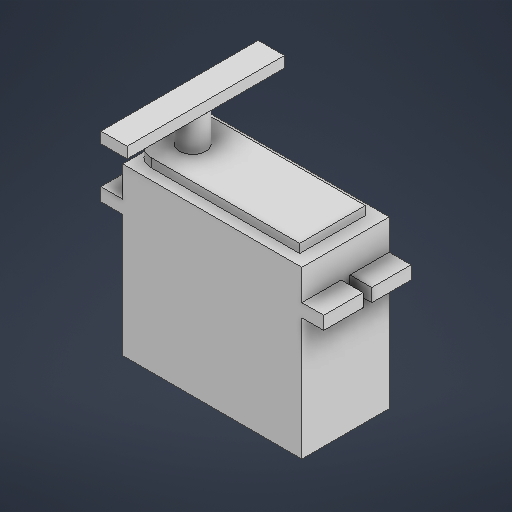
# Autodesk Inventor part: Servomoteur analogique FS5106B
Saved by Autodesk Inventor 2026.2 (Build 302298010, 298A)
## iProperties
Created: 2026-03-17
Part Number: Servomoteur analogique FS5106B
Material: Générique
Document SubType Name: Modeling
Designer: cleml
Density: 1 g/cm^3
Appearance: Par défaut
Author: cleml
Autodesk Inventor part; units mm, degrees
ref_plane "YZ Plane" through (0, 0, 0) normal (1, 0, 0) x (0, 1, 0)
ref_plane "XZ Plane" through (0, 0, 0) normal (0, 1, 0) x (-1, 0, 0)
ref_plane "XY Plane" through (0, 0, 0) normal (0, 0, 1) x (1, 0, 0)
sketch "Esquisse1" plane through (0, 0, 0) normal (0, 0, 1) x (1, 0, 0)
  line L0 (0, 0) -> (41, 0)
  line L1 (41, 0) -> (41, 38)
  line L2 (41, 38) -> (0, 38)
  line L3 (0, 38) -> (0, 0)
  dimension "d0" = 41
  dimension "d1" = 38
  constraints: 8 end point, 2 parallel, 1 horizontal, 1 perpendicular
  measures "d0" distance of L1.end L2.end
  measures "d1" distance of L0.end L1.end
extrude "Extrusion1" add sketch "Esquisse1" along normal blind 20
sketch "Esquisse2" plane through (0, 38, 0) normal (0, 1, 0) x (1, 0, 0)
  line L0 (0, 0) -> (0, -20) projected
  line L1 (0, -10) -> (0, -15)
  line L2 (0, -15) -> (0, -6.5)
  line L3 (0, -10) -> (38, -10)
  line L4 (38, -10) -> (38, -2.5)
  line L5 (38, -2.5) -> (4, -2.5)
  line L6 (0, -2.5) -> (0, -10)
  line L7 (38, -10) -> (38, -17.5)
  line L8 (38, -17.5) -> (4, -17.5)
  line L9 (0, -13.5) -> (0, -10)
  arc A0 (0, -13.5) -> (4, -17.5) centre (4, -13.5) ccw
  arc A1 (4, -2.5) -> (0, -6.5) centre (4, -6.5) ccw
  point P0 (0, -5)
  point P1 (0, -17.5)
  point P2 (0, -2.5)
  point P3 (0, -17.5)
  point P4 (0, -13.5)
  dimension "d6" = 38
  dimension "d9" = 15
  dimension "d10" = 4
  dimension "d11" = 4
  constraints: 18 end point, 6 point on line, 4 point on circle, 4 tangent, 3 symmetric about line, 2 centre point, 2 parallel, 1 horizontal, 1 midpoint, 1 perpendicular
  measures "d6" distance of L6.start L4.end
  measures "d9" distance between parallel lines of L5 L8
  measures "d10" radius of A0
  measures "d11" radius of A1
extrude "Extrusion2" add sketch "Esquisse2" along normal blind 2
sketch "Esquisse3" plane through (0, 40, 0) normal (0, 1, 0) x (1, 0, 0)
  line L0 (4, -17.5) -> (38, -17.5) projected
  line L1 (0, -6.5) -> (0, -13.5) projected
  line L2 (2.9996, -7) -> (8.9996, -7)
  line L3 (8.9996, -7) -> (8.9996, -13)
  line L4 (8.9996, -13) -> (2.9996, -13)
  line L5 (2.9996, -13) -> (2.9996, -7)
  line L6 (2.9996, -7) -> (8.9996, -13) construction
  line L7 (8.9996, -7) -> (2.9996, -13) construction
  point P0 (0, 0)
  point P1 (5.9996, -10)
  dimension "d12" = 7.5
  dimension "d13" = 5.9996
  dimension "d14" = 6
  dimension "d15" = 6
  constraints: 12 end point, 2 midpoint, 2 parallel, 1 horizontal, 1 perpendicular
  measures "d12" distance from line of L0 point (6, -10)
  measures "d13" distance from line of L1 point (6, -10)
  measures "d14" distance of L3.end L4.end
  measures "d15" distance of L2.end L3.end
extrude "Extrusion3" add sketch "Esquisse3" along normal blind 10
sketch "Esquisse4" plane through (8.9996, 40, 7) normal (0, 0, -1) x (-1, 0, 0)
  line L0 (6, 10) -> (0, 10) projected
  line L1 (0, 10) -> (6, 10)
  line L2 (6, 10) -> (6, 7.5)
  line L3 (6, 7.5) -> (0, 7.5)
  line L4 (0, 7.5) -> (0, 10)
  point P0 (8.9996, -40)
  dimension "d18" = 6
  dimension "d19" = 2.5
  constraints: 8 end point, 2 parallel, 1 horizontal, 1 perpendicular
  measures "d18" distance of L2.end L3.end
  measures "d19" distance of L1.end L2.end
extrude "Extrusion4" add sketch "Esquisse4" along normal blind 15
sketch "Esquisse6" plane through (2.9996, 40, 13) normal (0, 0, 1) x (1, 0, 0)
  line L0 (0, 10) -> (6, 10) projected
  line L1 (0, 10) -> (6, 10)
  line L2 (6, 10) -> (6, 7.5)
  line L3 (6, 7.5) -> (0, 7.5)
  line L4 (0, 7.5) -> (0, 10)
  point P0 (-2.9996, -40)
  dimension "d22" = 6
  dimension "d23" = 2.5
  constraints: 8 end point, 2 parallel, 1 horizontal, 1 perpendicular
  measures "d22" distance of L2.end L3.end
  measures "d23" distance of L1.end L2.end
extrude "Extrusion5" add sketch "Esquisse6" along normal blind 15
fillet "Congé1" radius 3 4 edges at (2.9996, 43.75, 7) (2.9996, 43.75, 13) (8.9996, 43.75, 13) (8.9996, 43.75, 7)
sketch "Esquisse9" plane through (41, 0, 0) normal (1, 0, 0) x (0, 0, -1)
  line L0 (-20, 0) -> (-20, 38) projected
  line L1 (-20, 38) -> (-20, 31)
  line L2 (-20, 31) -> (-11, 31)
  line L3 (-11, 31) -> (-11, 28)
  line L4 (-11, 28) -> (-20, 28)
  line L5 (-20, 28) -> (-20, 31)
  line L6 (-11, 31) -> (-10, 31)
  line L7 (0, 31) -> (-9, 31)
  line L8 (-9, 31) -> (-9, 28)
  line L9 (-9, 28) -> (0, 28)
  line L10 (0, 28) -> (0, 31)
  point P0 (0, 0)
  dimension "d38" = 7
  dimension "d39" = 9
  dimension "d40" = 3
  dimension "d41" = 1
  constraints: 20 end point, 2 horizontal, 2 parallel, 1 perpendicular, 1 point on line
  measures "d38" distance of L0.end L1.end
  measures "d39" distance of L3.end L4.end
  measures "d40" distance of L2.end L3.end
  measures "d41" distance of L2.end L6.end
extrude "Extrusion9" add sketch "Esquisse9" along normal blind 5
sketch "Esquisse10" plane through (0, 0, 0) normal (-1, 0, 0) x (0, 0, 1)
  line L0 (0, 38) -> (0, 31)
  line L1 (0, 38) -> (0, 0) projected
  line L2 (0, 31) -> (9, 31)
  line L3 (9, 31) -> (9, 28)
  line L4 (9, 28) -> (0, 28)
  line L5 (0, 28) -> (0, 31)
  line L6 (9, 31) -> (10, 31)
  line L7 (10, 31) -> (10, 24.8436)
  line L8 (20, 31) -> (11, 31)
  line L9 (11, 31) -> (11, 28)
  line L10 (11, 28) -> (20, 28)
  line L11 (20, 28) -> (20, 31)
  dimension "d44" = 7
  dimension "d45" = 9
  dimension "d46" = 3
  dimension "d47" = 1
  constraints: 22 end point, 4 symmetric about line, 2 horizontal, 2 parallel, 2 perpendicular, 1 point on line
  measures "d44" distance of L0.start L0.end
  measures "d45" distance of L3.end L4.end
  measures "d46" distance of L2.end L3.end
  measures "d47" distance of L2.end L6.end
extrude "Extrusion10" add sketch "Esquisse10" along normal blind 5
